Autodesk Fusion 360 part; units mm, degrees
(part 7 of 15)
  arc A95 (-74.6061, -67.9864) -> (-74.325, -69.279) centre (-2.0032, -52.8695) ccw
  spline S95 degree 5 poles (-74.325, -69.279) (-74.3068, -69.2823) (-74.2706, -69.289) (-74.2162, -69.2989) (-74.1437, -69.3119) (-74.053, -69.3279) (-73.9624, -69.3436) (-73.8718, -69.359) (-73.7813, -69.3741) (-73.6907, -69.3889) (-73.6002, -69.4033) (-73.5096, -69.4175) (-73.4191, -69.4313) (-73.3287, -69.4448) (-73.2382, -69.458) (-73.1478, -69.4709) (-73.0573, -69.4835) (-72.9669, -69.4957) (-72.8766, -69.5076) (-72.7862, -69.5192) (-72.6959, -69.5304) (-72.6056, -69.5413) (-72.5153, -69.5519) (-72.4251, -69.5621) (-72.3349, -69.572) (-72.2447, -69.5815) (-72.1546, -69.5907) (-72.0644, -69.5996) (-71.9744, -69.6081) (-71.8843, -69.6162) (-71.7943, -69.6239) (-71.7043, -69.6313) (-71.6144, -69.6384) (-71.5245, -69.645) (-71.4347, -69.6513) (-71.3449, -69.6572) (-71.2551, -69.6627) (-71.1654, -69.6678) (-71.0757, -69.6725) (-70.9861, -69.6768) (-70.8965, -69.6808) (-70.807, -69.6843) (-70.7248, -69.6871) (-70.6606, -69.689) (-70.6143, -69.6903) (-70.5859, -69.691) (-70.5753, -69.6913) knots -1 -1 -1 -1 -1 -1 -0.985714 -0.971429 -0.957143 -0.942857 -0.928571 -0.914286 -0.9 -0.885714 -0.871429 -0.857143 -0.842857 -0.828571 -0.814286 -0.8 -0.785714 -0.771429 -0.757143 -0.742857 -0.728571 -0.714286 -0.7 -0.685714 -0.671429 -0.657143 -0.642857 -0.628571 -0.614286 -0.6 -0.585714 -0.571429 -0.557143 -0.542857 -0.528571 -0.514286 -0.5 -0.485714 -0.471429 -0.457143 -0.442857 -0.428571 -0.414286 -0.405839 -0.405839 -0.405839 -0.405839 -0.405839 -0.405839
  arc A96 (-70.5753, -69.6913) -> (-70.2493, -70.9684) centre (-2.0032, -52.8695) ccw
  spline S96 degree 5 poles (-70.2493, -70.9684) (-70.2585, -70.9737) (-70.2831, -70.988) (-70.3231, -71.0113) (-70.3786, -71.0438) (-70.4493, -71.0856) (-70.5262, -71.1316) (-70.6029, -71.178) (-70.6795, -71.2247) (-70.756, -71.2718) (-70.8323, -71.3193) (-70.9084, -71.3672) (-70.9844, -71.4154) (-71.0603, -71.464) (-71.136, -71.5129) (-71.2115, -71.5621) (-71.287, -71.6118) (-71.3622, -71.6617) (-71.4374, -71.712) (-71.5124, -71.7626) (-71.5872, -71.8135) (-71.6619, -71.8648) (-71.7365, -71.9164) (-71.8109, -71.9683) (-71.8852, -72.0205) (-71.9594, -72.0731) (-72.0334, -72.1259) (-72.1073, -72.1791) (-72.1811, -72.2325) (-72.2547, -72.2863) (-72.3282, -72.3404) (-72.4015, -72.3947) (-72.4747, -72.4494) (-72.5478, -72.5043) (-72.6207, -72.5595) (-72.6935, -72.615) (-72.7662, -72.6709) (-72.8387, -72.7269) (-72.9111, -72.7833) (-72.9834, -72.8399) (-73.0555, -72.8969) (-73.1275, -72.9541) (-73.1994, -73.0115) (-73.2568, -73.0577) (-73.2998, -73.0925) (-73.3284, -73.1157) (-73.3427, -73.1273) knots 0.405839 0.405839 0.405839 0.405839 0.405839 0.405839 0.414286 0.428571 0.442857 0.457143 0.471429 0.485714 0.5 0.514286 0.528571 0.542857 0.557143 0.571429 0.585714 0.6 0.614286 0.628571 0.642857 0.657143 0.671429 0.685714 0.7 0.714286 0.728571 0.742857 0.757143 0.771429 0.785714 0.8 0.814286 0.828571 0.842857 0.857143 0.871429 0.885714 0.9 0.914286 0.928571 0.942857 0.957143 0.971429 0.985714 1 1 1 1 1 1
  arc A97 (-73.3427, -73.1273) -> (-72.97, -74.3965) centre (-2.0032, -52.8695) ccw
  spline S97 degree 5 poles (-72.97, -74.3965) (-72.9517, -74.3986) (-72.9151, -74.4026) (-72.8601, -74.4087) (-72.7869, -74.4165) (-72.6953, -74.426) (-72.6038, -74.4352) (-72.5124, -74.444) (-72.421, -74.4526) (-72.3296, -74.4609) (-72.2382, -74.4689) (-72.1469, -74.4765) (-72.0557, -74.4839) (-71.9645, -74.4909) (-71.8733, -74.4976) (-71.7822, -74.504) (-71.6911, -74.5101) (-71.6, -74.5158) (-71.509, -74.5213) (-71.4181, -74.5264) (-71.3272, -74.5311) (-71.2364, -74.5356) (-71.1456, -74.5397) (-71.0548, -74.5434) (-70.9641, -74.5469) (-70.8735, -74.5499) (-70.7829, -74.5527) (-70.6924, -74.5551) (-70.602, -74.5571) (-70.5116, -74.5588) (-70.4212, -74.5601) (-70.331, -74.5611) (-70.2408, -74.5616) (-70.1506, -74.5619) (-70.0606, -74.5617) (-69.9706, -74.5612) (-69.8806, -74.5603) (-69.7908, -74.559) (-69.701, -74.5573) (-69.6113, -74.5552) (-69.5217, -74.5527) (-69.4321, -74.5498) (-69.35, -74.5468) (-69.2858, -74.5441) (-69.2395, -74.5421) (-69.2111, -74.5408) (-69.2005, -74.5403) knots -1 -1 -1 -1 -1 -1 -0.985714 -0.971429 -0.957143 -0.942857 -0.928571 -0.914286 -0.9 -0.885714 -0.871429 -0.857143 -0.842857 -0.828571 -0.814286 -0.8 -0.785714 -0.771429 -0.757143 -0.742857 -0.728571 -0.714286 -0.7 -0.685714 -0.671429 -0.657143 -0.642857 -0.628571 -0.614286 -0.6 -0.585714 -0.571429 -0.557143 -0.542857 -0.528571 -0.514286 -0.5 -0.485714 -0.471429 -0.457143 -0.442857 -0.428571 -0.414286 -0.405839 -0.405839 -0.405839 -0.405839 -0.405839 -0.405839
  arc A98 (-69.2005, -74.5403) -> (-68.7843, -75.791) centre (-2.0032, -52.8695) ccw
  spline S98 degree 5 poles (-68.7843, -75.791) (-68.793, -75.7969) (-68.8166, -75.8129) (-68.8548, -75.839) (-68.9078, -75.8753) (-68.9754, -75.9221) (-69.0488, -75.9735) (-69.1221, -76.0252) (-69.1951, -76.0773) (-69.268, -76.1297) (-69.3407, -76.1825) (-69.4132, -76.2357) (-69.4856, -76.2892) (-69.5578, -76.3431) (-69.6298, -76.3973) (-69.7017, -76.4518) (-69.7734, -76.5066) (-69.8449, -76.5618) (-69.9163, -76.6174) (-69.9874, -76.6732) (-70.0585, -76.7293) (-70.1293, -76.7858) (-70.2, -76.8426) (-70.2706, -76.8997) (-70.341, -76.9571) (-70.4112, -77.0148) (-70.4813, -77.0728) (-70.5512, -77.131) (-70.6209, -77.1896) (-70.6905, -77.2485) (-70.7599, -77.3077) (-70.8292, -77.3671) (-70.8983, -77.4269) (-70.9673, -77.4869) (-71.0361, -77.5472) (-71.1048, -77.6077) (-71.1733, -77.6686) (-71.2416, -77.7297) (-71.3098, -77.7911) (-71.3779, -77.8527) (-71.4458, -77.9146) (-71.5135, -77.9768) (-71.5811, -78.0393) (-71.635, -78.0894) (-71.6754, -78.1272) (-71.7023, -78.1524) (-71.7158, -78.165) knots 0.405839 0.405839 0.405839 0.405839 0.405839 0.405839 0.414286 0.428571 0.442857 0.457143 0.471429 0.485714 0.5 0.514286 0.528571 0.542857 0.557143 0.571429 0.585714 0.6 0.614286 0.628571 0.642857 0.657143 0.671429 0.685714 0.7 0.714286 0.728571 0.742857 0.757143 0.771429 0.785714 0.8 0.814286 0.828571 0.842857 0.857143 0.871429 0.885714 0.9 0.914286 0.928571 0.942857 0.957143 0.971429 0.985714 1 1 1 1 1 1
  arc A99 (-71.7158, -78.165) -> (-71.2535, -79.4044) centre (-2.0032, -52.8695) ccw
  spline S99 degree 5 poles (-71.2535, -79.4044) (-71.2351, -79.4051) (-71.1982, -79.4066) (-71.143, -79.4086) (-71.0694, -79.4112) (-70.9774, -79.4142) (-70.8855, -79.4168) (-70.7936, -79.4191) (-70.7018, -79.4212) (-70.6101, -79.4229) (-70.5184, -79.4243) (-70.4268, -79.4255) (-70.3352, -79.4263) (-70.2438, -79.4268) (-70.1523, -79.427) (-70.061, -79.4268) (-69.9697, -79.4264) (-69.8785, -79.4257) (-69.7873, -79.4246) (-69.6962, -79.4232) (-69.6052, -79.4214) (-69.5143, -79.4194) (-69.4235, -79.417) (-69.3327, -79.4143) (-69.242, -79.4112) (-69.1514, -79.4079) (-69.0608, -79.4041) (-68.9704, -79.4) (-68.88, -79.3956) (-68.7897, -79.3908) (-68.6995, -79.3857) (-68.6094, -79.3802) (-68.5194, -79.3744) (-68.4295, -79.3682) (-68.3397, -79.3616) (-68.2499, -79.3547) (-68.1603, -79.3473) (-68.0708, -79.3396) (-67.9813, -79.3315) (-67.892, -79.3231) (-67.8028, -79.3142) (-67.7137, -79.3049) (-67.632, -79.296) (-67.5681, -79.2888) (-67.5221, -79.2835) (-67.4938, -79.2801) (-67.4833, -79.2789) knots -1 -1 -1 -1 -1 -1 -0.985714 -0.971429 -0.957143 -0.942857 -0.928571 -0.914286 -0.9 -0.885714 -0.871429 -0.857143 -0.842857 -0.828571 -0.814286 -0.8 -0.785714 -0.771429 -0.757143 -0.742857 -0.728571 -0.714286 -0.7 -0.685714 -0.671429 -0.657143 -0.642857 -0.628571 -0.614286 -0.6 -0.585714 -0.571429 -0.557143 -0.542857 -0.528571 -0.514286 -0.5 -0.485714 -0.471429 -0.457143 -0.442857 -0.428571 -0.414286 -0.405839 -0.405839 -0.405839 -0.405839 -0.405839 -0.405839
  arc A100 (-67.4833, -79.2789) -> (-66.9789, -80.4967) centre (-2.0032, -52.8695) ccw
  spline S100 degree 5 poles (-66.9789, -80.4967) (-66.9872, -80.5032) (-67.0096, -80.5208) (-67.0459, -80.5496) (-67.0961, -80.5896) (-67.1602, -80.6411) (-67.2298, -80.6976) (-67.2991, -80.7544) (-67.3683, -80.8116) (-67.4372, -80.8691) (-67.506, -80.9269) (-67.5746, -80.9851) (-67.6429, -81.0437) (-67.7111, -81.1025) (-67.7791, -81.1617) (-67.8469, -81.2213) (-67.9144, -81.2811) (-67.9818, -81.3412) (-68.0491, -81.4017) (-68.1161, -81.4625) (-68.1829, -81.5236) (-68.2496, -81.5849) (-68.3161, -81.6466) (-68.3824, -81.7086) (-68.4485, -81.7709) (-68.5144, -81.8334) (-68.5801, -81.8963) (-68.6457, -81.9594) (-68.7111, -82.0228) (-68.7763, -82.0865) (-68.8414, -82.1505) (-68.9062, -82.2147) (-68.9709, -82.2792) (-69.0354, -82.344) (-69.0997, -82.409) (-69.1639, -82.4743) (-69.2279, -82.5399) (-69.2917, -82.6058) (-69.3553, -82.6719) (-69.4188, -82.7382) (-69.4821, -82.8048) (-69.5453, -82.8717) (-69.6082, -82.9388) (-69.6585, -82.9927) (-69.6961, -83.0332) (-69.7211, -83.0603) (-69.7336, -83.0738) knots 0.405839 0.405839 0.405839 0.405839 0.405839 0.405839 0.414286 0.428571 0.442857 0.457143 0.471429 0.485714 0.5 0.514286 0.528571 0.542857 0.557143 0.571429 0.585714 0.6 0.614286 0.628571 0.642857 0.657143 0.671429 0.685714 0.7 0.714286 0.728571 0.742857 0.757143 0.771429 0.785714 0.8 0.814286 0.828571 0.842857 0.857143 0.871429 0.885714 0.9 0.914286 0.928571 0.942857 0.957143 0.971429 0.985714 1 1 1 1 1 1
  arc A101 (-69.7336, -83.0738) -> (-69.1841, -84.2771) centre (-2.0032, -52.8695) ccw
  spline S101 degree 5 poles (-69.1841, -84.2771) (-69.1657, -84.2765) (-69.1288, -84.2753) (-69.0736, -84.2734) (-68.9999, -84.2707) (-68.908, -84.2671) (-68.8161, -84.2632) (-68.7243, -84.2589) (-68.6326, -84.2544) (-68.541, -84.2496) (-68.4494, -84.2445) (-68.358, -84.2391) (-68.2666, -84.2334) (-68.1753, -84.2273) (-68.0841, -84.221) (-67.993, -84.2144) (-67.902, -84.2074) (-67.811, -84.2002) (-67.7202, -84.1926) (-67.6295, -84.1847) (-67.5388, -84.1765) (-67.4483, -84.1679) (-67.3578, -84.1591) (-67.2675, -84.1499) (-67.1772, -84.1404) (-67.0871, -84.1305) (-66.997, -84.1203) (-66.9071, -84.1098) (-66.8173, -84.099) (-66.7276, -84.0878) (-66.638, -84.0762) (-66.5485, -84.0643) (-66.4591, -84.0521) (-66.3698, -84.0395) (-66.2807, -84.0265) (-66.1917, -84.0132) (-66.1028, -83.9995) (-66.0141, -83.9854) (-65.9254, -83.9709) (-65.837, -83.9561) (-65.7486, -83.9409) (-65.6604, -83.9253) (-65.5795, -83.9106) (-65.5163, -83.8988) (-65.4708, -83.8902) (-65.4429, -83.8849) (-65.4325, -83.8829) knots -1 -1 -1 -1 -1 -1 -0.985714 -0.971429 -0.957143 -0.942857 -0.928571 -0.914286 -0.9 -0.885714 -0.871429 -0.857143 -0.842857 -0.828571 -0.814286 -0.8 -0.785714 -0.771429 -0.757143 -0.742857 -0.728571 -0.714286 -0.7 -0.685714 -0.671429 -0.657143 -0.642857 -0.628571 -0.614286 -0.6 -0.585714 -0.571429 -0.557143 -0.542857 -0.528571 -0.514286 -0.5 -0.485714 -0.471429 -0.457143 -0.442857 -0.428571 -0.414286 -0.405839 -0.405839 -0.405839 -0.405839 -0.405839 -0.405839
  arc A102 (-65.4325, -83.8829) -> (-64.8425, -85.0616) centre (-2.0032, -52.8695) ccw
  spline S102 degree 5 poles (-64.8425, -85.0616) (-64.8503, -85.0687) (-64.8713, -85.0879) (-64.9055, -85.1191) (-64.9528, -85.1627) (-65.013, -85.2186) (-65.0783, -85.2799) (-65.1435, -85.3415) (-65.2084, -85.4035) (-65.2731, -85.4657) (-65.3375, -85.5284) (-65.4017, -85.5913) (-65.4658, -85.6546) (-65.5296, -85.7181) (-65.5931, -85.782) (-65.6565, -85.8462) (-65.7197, -85.9108) (-65.7826, -85.9756) (-65.8453, -86.0407) (-65.9078, -86.1061) (-65.9702, -86.1718) (-66.0323, -86.2377) (-66.0942, -86.304) (-66.1559, -86.3705) (-66.2174, -86.4374) (-66.2787, -86.5045) (-66.3398, -86.5718) (-66.4007, -86.6395) (-66.4614, -86.7074) (-66.5219, -86.7756) (-66.5822, -86.844) (-66.6423, -86.9127) (-66.7022, -86.9817) (-66.7619, -87.0509) (-66.8215, -87.1204) (-66.8808, -87.1901) (-66.9399, -87.2601) (-66.9989, -87.3303) (-67.0577, -87.4008) (-67.1162, -87.4715) (-67.1746, -87.5424) (-67.2328, -87.6136) (-67.2908, -87.6851) (-67.3371, -87.7424) (-67.3717, -87.7855) (-67.3948, -87.8143) (-67.4063, -87.8287) knots 0.405839 0.405839 0.405839 0.405839 0.405839 0.405839 0.414286 0.428571 0.442857 0.457143 0.471429 0.485714 0.5 0.514286 0.528571 0.542857 0.557143 0.571429 0.585714 0.6 0.614286 0.628571 0.642857 0.657143 0.671429 0.685714 0.7 0.714286 0.728571 0.742857 0.757143 0.771429 0.785714 0.8 0.814286 0.828571 0.842857 0.857143 0.871429 0.885714 0.9 0.914286 0.928571 0.942857 0.957143 0.971429 0.985714 1 1 1 1 1 1
  arc A103 (-67.4063, -87.8287) -> (-66.7723, -88.9897) centre (-2.0032, -52.8695) ccw
  spline S103 degree 5 poles (-66.7723, -88.9897) (-66.754, -88.9878) (-66.7173, -88.9839) (-66.6623, -88.9781) (-66.5891, -88.9702) (-66.4976, -88.96) (-66.4063, -88.9496) (-66.315, -88.9388) (-66.2239, -88.9277) (-66.1328, -88.9164) (-66.0419, -88.9048) (-65.951, -88.8928) (-65.8603, -88.8806) (-65.7697, -88.8681) (-65.6791, -88.8553) (-65.5887, -88.8422) (-65.4984, -88.8287) (-65.4083, -88.815) (-65.3182, -88.801) (-65.2282, -88.7866) (-65.1384, -88.772) (-65.0487, -88.757) (-64.9591, -88.7417) (-64.8697, -88.7261) (-64.7803, -88.7102) (-64.6911, -88.6939) (-64.602, -88.6773) (-64.5131, -88.6604) (-64.4242, -88.6432) (-64.3356, -88.6256) (-64.247, -88.6077) (-64.1586, -88.5894) (-64.0703, -88.5709) (-63.9822, -88.5519) (-63.8942, -88.5326) (-63.8064, -88.513) (-63.7187, -88.493) (-63.6312, -88.4726) (-63.5438, -88.4519) (-63.4566, -88.4307) (-63.3696, -88.4093) (-63.2827, -88.3874) (-63.2031, -88.367) (-63.1409, -88.3508) (-63.0961, -88.3389) (-63.0686, -88.3316) (-63.0584, -88.3289) knots -1 -1 -1 -1 -1 -1 -0.985714 -0.971429 -0.957143 -0.942857 -0.928571 -0.914286 -0.9 -0.885714 -0.871429 -0.857143 -0.842857 -0.828571 -0.814286 -0.8 -0.785714 -0.771429 -0.757143 -0.742857 -0.728571 -0.714286 -0.7 -0.685714 -0.671429 -0.657143 -0.642857 -0.628571 -0.614286 -0.6 -0.585714 -0.571429 -0.557143 -0.542857 -0.528571 -0.514286 -0.5 -0.485714 -0.471429 -0.457143 -0.442857 -0.428571 -0.414286 -0.405839 -0.405839 -0.405839 -0.405839 -0.405839 -0.405839
  arc A104 (-63.0584, -88.3289) -> (-62.3858, -89.4625) centre (-2.0032, -52.8695) ccw
  spline S104 degree 5 poles (-62.3858, -89.4625) (-62.3931, -89.4701) (-62.4127, -89.4907) (-62.4446, -89.5244) (-62.4886, -89.5712) (-62.5447, -89.6313) (-62.6055, -89.697) (-62.6661, -89.7631) (-62.7264, -89.8296) (-62.7865, -89.8963) (-62.8463, -89.9634) (-62.9059, -90.0307) (-62.9652, -90.0984) (-63.0243, -90.1664) (-63.0832, -90.2346) (-63.1418, -90.3032) (-63.2002, -90.372) (-63.2583, -90.4412) (-63.3163, -90.5106) (-63.374, -90.5803) (-63.4314, -90.6503) (-63.4887, -90.7205) (-63.5457, -90.791) (-63.6025, -90.8618) (-63.6591, -90.9328) (-63.7154, -91.0041) (-63.7715, -91.0757) (-63.8275, -91.1475) (-63.8832, -91.2196) (-63.9386, -91.2919) (-63.9939, -91.3645) (-64.049, -91.4373) (-64.1038, -91.5103) (-64.1585, -91.5837) (-64.2129, -91.6572) (-64.2671, -91.731) (-64.3211, -91.805) (-64.3749, -91.8792) (-64.4285, -91.9537) (-64.4819, -92.0284) (-64.535, -92.1034) (-64.588, -92.1785) (-64.6408, -92.2539) (-64.6828, -92.3144) (-64.7143, -92.3599) (-64.7352, -92.3902) (-64.7457, -92.4054) knots 0.405839 0.405839 0.405839 0.405839 0.405839 0.405839 0.414286 0.428571 0.442857 0.457143 0.471429 0.485714 0.5 0.514286 0.528571 0.542857 0.557143 0.571429 0.585714 0.6 0.614286 0.628571 0.642857 0.657143 0.671429 0.685714 0.7 0.714286 0.728571 0.742857 0.757143 0.771429 0.785714 0.8 0.814286 0.828571 0.842857 0.857143 0.871429 0.885714 0.9 0.914286 0.928571 0.942857 0.957143 0.971429 0.985714 1 1 1 1 1 1
  arc A105 (-64.7457, -92.4054) -> (-64.0305, -93.5182) centre (-2.0032, -52.8695) ccw
  spline S105 degree 5 poles (-64.0305, -93.5182) (-64.0124, -93.515) (-63.9761, -93.5086) (-63.9216, -93.4989) (-63.8491, -93.4857) (-63.7586, -93.4691) (-63.6683, -93.4521) (-63.578, -93.4348) (-63.4879, -93.4173) (-63.3979, -93.3995) (-63.308, -93.3814) (-63.2182, -93.363) (-63.1286, -93.3444) (-63.0391, -93.3254) (-62.9497, -93.3062) (-62.8605, -93.2866) (-62.7714, -93.2668) (-62.6824, -93.2467) (-62.5936, -93.2263) (-62.5049, -93.2055) (-62.4163, -93.1845) (-62.3279, -93.1632) (-62.2396, -93.1415) (-62.1515, -93.1196) (-62.0635, -93.0973) (-61.9757, -93.0747) (-61.888, -93.0518) (-61.8005, -93.0286) (-61.7131, -93.0051) (-61.6259, -92.9812) (-61.5389, -92.9571) (-61.452, -92.9325) (-61.3653, -92.9077) (-61.2787, -92.8825) (-61.1924, -92.857) (-61.1062, -92.8311) (-61.0201, -92.8049) (-60.9343, -92.7784) (-60.8486, -92.7515) (-60.7631, -92.7242) (-60.6778, -92.6965) (-60.5927, -92.6685) (-60.5148, -92.6425) (-60.4539, -92.6219) (-60.4101, -92.6069) (-60.3832, -92.5976) (-60.3732, -92.5941) knots -1 -1 -1 -1 -1 -1 -0.985714 -0.971429 -0.957143 -0.942857 -0.928571 -0.914286 -0.9 -0.885714 -0.871429 -0.857143 -0.842857 -0.828571 -0.814286 -0.8 -0.785714 -0.771429 -0.757143 -0.742857 -0.728571 -0.714286 -0.7 -0.685714 -0.671429 -0.657143 -0.642857 -0.628571 -0.614286 -0.6 -0.585714 -0.571429 -0.557143 -0.542857 -0.528571 -0.514286 -0.5 -0.485714 -0.471429 -0.457143 -0.442857 -0.428571 -0.414286 -0.405839 -0.405839 -0.405839 -0.405839 -0.405839 -0.405839
  arc A106 (-60.3732, -92.5941) -> (-59.6214, -93.6769) centre (-2.0032, -52.8695) ccw
  spline S106 degree 5 poles (-59.6214, -93.6769) (-59.6282, -93.685) (-59.6462, -93.707) (-59.6756, -93.7428) (-59.7162, -93.7926) (-59.7679, -93.8566) (-59.8238, -93.9265) (-59.8795, -93.9968) (-59.935, -94.0673) (-59.9901, -94.1382) (-60.045, -94.2093) (-60.0996, -94.2808) (-60.154, -94.3525) (-60.2081, -94.4245) (-60.2619, -94.4968) (-60.3155, -94.5694) (-60.3688, -94.6422) (-60.4219, -94.7153) (-60.4747, -94.7887) (-60.5273, -94.8623) (-60.5797, -94.9362) (-60.6317, -95.0104) (-60.6836, -95.0848) (-60.7352, -95.1594) (-60.7866, -95.2343) (-60.8377, -95.3095) (-60.8886, -95.3849) (-60.9392, -95.4605) (-60.9896, -95.5363) (-61.0398, -95.6124) (-61.0898, -95.6888) (-61.1395, -95.7653) (-61.189, -95.8421) (-61.2383, -95.9191) (-61.2873, -95.9964) (-61.3361, -96.0738) (-61.3847, -96.1515) (-61.4331, -96.2294) (-61.4812, -96.3075) (-61.5291, -96.3858) (-61.5768, -96.4644) (-61.6243, -96.5431) (-61.6715, -96.6221) (-61.7092, -96.6854) (-61.7373, -96.733) (-61.756, -96.7648) (-61.7653, -96.7807) knots 0.405839 0.405839 0.405839 0.405839 0.405839 0.405839 0.414286 0.428571 0.442857 0.457143 0.471429 0.485714 0.5 0.514286 0.528571 0.542857 0.557143 0.571429 0.585714 0.6 0.614286 0.628571 0.642857 0.657143 0.671429 0.685714 0.7 0.714286 0.728571 0.742857 0.757143 0.771429 0.785714 0.8 0.814286 0.828571 0.842857 0.857143 0.871429 0.885714 0.9 0.914286 0.928571 0.942857 0.957143 0.971429 0.985714 1 1 1 1 1 1
  arc A107 (-61.7653, -96.7807) -> (-60.9726, -97.8396) centre (-2.0032, -52.8695) ccw
  spline S107 degree 5 poles (-60.9726, -97.8396) (-60.9548, -97.8351) (-60.919, -97.8261) (-60.8654, -97.8126) (-60.794, -97.7943) (-60.705, -97.7712) (-60.616, -97.7478) (-60.5272, -97.7242) (-60.4386, -97.7003) (-60.3501, -97.6761) (-60.2617, -97.6516) (-60.1735, -97.6269) (-60.0854, -97.6019) (-59.9975, -97.5766) (-59.9097, -97.551) (-59.8221, -97.5252) (-59.7346, -97.499) (-59.6473, -97.4726) (-59.5602, -97.4459) (-59.4732, -97.4189) (-59.3863, -97.3916) (-59.2997, -97.364) (-59.2132, -97.3361) (-59.1268, -97.3079) (-59.0407, -97.2795) (-58.9547, -97.2507) (-58.8689, -97.2216) (-58.7832, -97.1922) (-58.6978, -97.1625) (-58.6125, -97.1325) (-58.5274, -97.1021) (-58.4425, -97.0715) (-58.3577, -97.0405) (-58.2732, -97.0092) (-58.1889, -96.9776) (-58.1047, -96.9457) (-58.0208, -96.9134) (-57.9371, -96.8808) (-57.8535, -96.8478) (-57.7702, -96.8145) (-57.6871, -96.7809) (-57.6042, -96.7469) (-57.5283, -96.7153) (-57.4691, -96.6904) (-57.4264, -96.6723) (-57.4003, -96.6611) (-57.3905, -96.657) knots -1 -1 -1 -1 -1 -1 -0.985714 -0.971429 -0.957143 -0.942857 -0.928571 -0.914286 -0.9 -0.885714 -0.871429 -0.857143 -0.842857 -0.828571 -0.814286 -0.8 -0.785714 -0.771429 -0.757143 -0.742857 -0.728571 -0.714286 -0.7 -0.685714 -0.671429 -0.657143 -0.642857 -0.628571 -0.614286 -0.6 -0.585714 -0.571429 -0.557143 -0.542857 -0.528571 -0.514286 -0.5 -0.485714 -0.471429 -0.457143 -0.442857 -0.428571 -0.414286 -0.405839 -0.405839 -0.405839 -0.405839 -0.405839 -0.405839
  arc A108 (-57.3905, -96.657) -> (-56.5635, -97.6833) centre (-2.0032, -52.8695) ccw
  spline S108 degree 5 poles (-56.5635, -97.6833) (-56.5696, -97.6919) (-56.5861, -97.7151) (-56.6128, -97.753) (-56.6497, -97.8056) (-56.6967, -97.873) (-56.7476, -97.9468) (-56.7981, -98.0208) (-56.8484, -98.0952) (-56.8983, -98.1698) (-56.948, -98.2447) (-56.9974, -98.3198) (-57.0465, -98.3953) (-57.0953, -98.4709) (-57.1438, -98.5469) (-57.1921, -98.6231) (-57.2401, -98.6996) (-57.2878, -98.7763) (-57.3353, -98.8532) (-57.3825, -98.9304) (-57.4294, -99.0078) (-57.4761, -99.0855) (-57.5225, -99.1634) (-57.5686, -99.2416) (-57.6145, -99.3199) (-57.6601, -99.3985) (-57.7055, -99.4774) (-57.7507, -99.5564) (-57.7955, -99.6357) (-57.8402, -99.7152) (-57.8845, -99.7948) (-57.9287, -99.8748) (-57.9726, -99.9549) (-58.0162, -100.0352) (-58.0596, -100.1157) (-58.1028, -100.1965) (-58.1457, -100.2774) (-58.1884, -100.3586) (-58.2308, -100.4399) (-58.273, -100.5215) (-58.315, -100.6032) (-58.3567, -100.6852) (-58.3982, -100.7673) (-58.4313, -100.8331) (-58.4559, -100.8826) (-58.4723, -100.9157) (-58.4805, -100.9322) knots 0.405839 0.405839 0.405839 0.405839 0.405839 0.405839 0.414286 0.428571 0.442857 0.457143 0.471429 0.485714 0.5 0.514286 0.528571 0.542857 0.557143 0.571429 0.585714 0.6 0.614286 0.628571 0.642857 0.657143 0.671429 0.685714 0.7 0.714286 0.728571 0.742857 0.757143 0.771429 0.785714 0.8 0.814286 0.828571 0.842857 0.857143 0.871429 0.885714 0.9 0.914286 0.928571 0.942857 0.957143 0.971429 0.985714 1 1 1 1 1 1
  arc A109 (-58.4805, -100.9322) -> (-57.6143, -101.9319) centre (-2.0032, -52.8695) ccw
  spline S109 degree 5 poles (-57.6143, -101.9319) (-57.5967, -101.9261) (-57.5617, -101.9146) (-57.5092, -101.8972) (-57.4393, -101.8739) (-57.3521, -101.8445) (-57.2651, -101.8149) (-57.1782, -101.785) (-57.0915, -101.7548) (-57.0049, -101.7243) (-56.9185, -101.6936) (-56.8323, -101.6627) (-56.7462, -101.6315) (-56.6603, -101.6) (-56.5746, -101.5682) (-56.4891, -101.5361) (-56.4037, -101.5038) (-56.3185, -101.4712) (-56.2335, -101.4384) (-56.1486, -101.4052) (-56.064, -101.3718) (-55.9795, -101.3381) (-55.8952, -101.3041) (-55.8111, -101.2699) (-55.7272, -101.2353) (-55.6435, -101.2005) (-55.5599, -101.1653) (-55.4766, -101.1299) (-55.3935, -101.0942) (-55.3106, -101.0582) (-55.2278, -101.0218) (-55.1453, -100.9852) (-55.063, -100.9483) (-54.9809, -100.911) (-54.8991, -100.8735) (-54.8174, -100.8356) (-54.736, -100.7974) (-54.6548, -100.7589) (-54.5739, -100.7201) (-54.4931, -100.6809) (-54.4126, -100.6414) (-54.3324, -100.6016) (-54.2589, -100.5647) (-54.2016, -100.5356) (-54.1604, -100.5146) (-54.1351, -100.5016) (-54.1257, -100.4967) knots -1 -1 -1 -1 -1 -1 -0.985714 -0.971429 -0.957143 -0.942857 -0.928571 -0.914286 -0.9 -0.885714 -0.871429 -0.857143 -0.842857 -0.828571 -0.814286 -0.8 -0.785714 -0.771429 -0.757143 -0.742857 -0.728571 -0.714286 -0.7 -0.685714 -0.671429 -0.657143 -0.642857 -0.628571 -0.614286 -0.6 -0.585714 -0.571429 -0.557143 -0.542857 -0.528571 -0.514286 -0.5 -0.485714 -0.471429 -0.457143 -0.442857 -0.428571 -0.414286 -0.405839 -0.405839 -0.405839 -0.405839 -0.405839 -0.405839
  arc A110 (-54.1257, -100.4967) -> (-53.2275, -101.4614) centre (-2.0032, -52.8695) ccw
  spline S110 degree 5 poles (-53.2275, -101.4614) (-53.233, -101.4705) (-53.2477, -101.4948) (-53.2717, -101.5344) (-53.3048, -101.5895) (-53.3468, -101.6602) (-53.3923, -101.7374) (-53.4374, -101.8148) (-53.4822, -101.8926) (-53.5268, -101.9705) (-53.571, -102.0488) (-53.6149, -102.1273) (-53.6585, -102.206) (-53.7018, -102.285) (-53.7448, -102.3642) (-53.7875, -102.4437) (-53.8299, -102.5233) (-53.872, -102.6033) (-53.9139, -102.6834) (-53.9554, -102.7638) (-53.9967, -102.8444) (-54.0377, -102.9252) (-54.0784, -103.0062) (-54.1189, -103.0874) (-54.1591, -103.1689) (-54.199, -103.2505) (-54.2386, -103.3324) (-54.278, -103.4144) (-54.3171, -103.4967) (-54.356, -103.5792) (-54.3945, -103.6618) (-54.4329, -103.7447) (-54.4709, -103.8277) (-54.5087, -103.911) (-54.5463, -103.9944) (-54.5836, -104.078) (-54.6206, -104.1618) (-54.6574, -104.2458) (-54.6939, -104.33) (-54.7302, -104.4143) (-54.7662, -104.4988) (-54.802, -104.5835) (-54.8376, -104.6684) (-54.8658, -104.7365) (-54.8869, -104.7876) (-54.9009, -104.8217) (-54.9078, -104.8388) knots 0.405839 0.405839 0.405839 0.405839 0.405839 0.405839 0.414286 0.428571 0.442857 0.457143 0.471429 0.485714 0.5 0.514286 0.528571 0.542857 0.557143 0.571429 0.585714 0.6 0.614286 0.628571 0.642857 0.657143 0.671429 0.685714 0.7 0.714286 0.728571 0.742857 0.757143 0.771429 0.785714 0.8 0.814286 0.828571 0.842857 0.857143 0.871429 0.885714 0.9 0.914286 0.928571 0.942857 0.957143 0.971429 0.985714 1 1 1 1 1 1
  arc A111 (-54.9078, -104.8388) -> (-53.9725, -105.7741) centre (-2.0032, -52.8695) ccw
  spline S111 degree 5 poles (-53.9725, -105.7741) (-53.9554, -105.7671) (-53.9213, -105.7531) (-53.8702, -105.7321) (-53.8022, -105.7038) (-53.7173, -105.6683) (-53.6326, -105.6325) (-53.548, -105.5965) (-53.4637, -105.5602) (-53.3795, -105.5236) (-53.2955, -105.4869) (-53.2117, -105.4498) (-53.1281, -105.4125) (-53.0447, -105.375) (-52.9615, -105.3372) (-52.8784, -105.2991) (-52.7955, -105.2608) (-52.7129, -105.2222) (-52.6304, -105.1834) (-52.5482, -105.1443) (-52.4661, -105.1049) (-52.3842, -105.0653) (-52.3026, -105.0253) (-52.2211, -104.9852) (-52.1399, -104.9447) (-52.0589, -104.904) (-51.9781, -104.863) (-51.8975, -104.8217) (-51.8171, -104.7801) (-51.737, -104.7383) (-51.6571, -104.6962) (-51.5774, -104.6537) (-51.4979, -104.611) (-51.4187, -104.568) (-51.3397, -104.5247) (-51.261, -104.4811) (-51.1825, -104.4372) (-51.1043, -104.393) (-51.0263, -104.3485) (-50.9486, -104.3037) (-50.8711, -104.2586) (-50.7939, -104.2131) (-50.7232, -104.1711) (-50.6682, -104.138) (-50.6285, -104.114) (-50.6042, -104.0992) (-50.5952, -104.0937) knots -1 -1 -1 -1 -1 -1 -0.985714 -0.971429 -0.957143 -0.942857 -0.928571 -0.914286 -0.9 -0.885714 -0.871429 -0.857143 -0.842857 -0.828571 -0.814286 -0.8 -0.785714 -0.771429 -0.757143 -0.742857 -0.728571 -0.714286 -0.7 -0.685714 -0.671429 -0.657143 -0.642857 -0.628571 -0.614286 -0.6 -0.585714 -0.571429 -0.557143 -0.542857 -0.528571 -0.514286 -0.5 -0.485714 -0.471429 -0.457143 -0.442857 -0.428571 -0.414286 -0.405839 -0.405839 -0.405839 -0.405839 -0.405839 -0.405839
  arc A112 (-50.5952, -104.0937) -> (-49.6305, -104.9919) centre (-2.0032, -52.8695) ccw
  spline S112 degree 5 poles (-49.6305, -104.9919) (-49.6353, -105.0013) (-49.6483, -105.0266) (-49.6694, -105.0679) (-49.6985, -105.1252) (-49.7353, -105.1987) (-49.7752, -105.2789) (-49.8147, -105.3594) (-49.8538, -105.4401) (-49.8927, -105.5211) (-49.9312, -105.6023) (-49.9693, -105.6837) (-50.0072, -105.7653) (-50.0448, -105.8472) (-50.082, -105.9293) (-50.1189, -106.0116) (-50.1556, -106.0941) (-50.1919, -106.1768) (-50.2279, -106.2597) (-50.2636, -106.3429) (-50.2991, -106.4262) (-50.3342, -106.5097) (-50.3691, -106.5934) (-50.4036, -106.6774) (-50.4379, -106.7615) (-50.4719, -106.8457) (-50.5056, -106.9302) (-50.539, -107.0149) (-50.5721, -107.0997) (-50.605, -107.1848) (-50.6376, -107.27) (-50.6699, -107.3553) (-50.7019, -107.4409) (-50.7337, -107.5266) (-50.7652, -107.6125) (-50.7964, -107.6986) (-50.8274, -107.7848) (-50.8581, -107.8712) (-50.8885, -107.9578) (-50.9187, -108.0445) (-50.9486, -108.1314) (-50.9783, -108.2184) (-51.0077, -108.3056) (-51.031, -108.3755) (-51.0483, -108.428) (-51.0598, -108.463) (-51.0656, -108.4805) knots 0.405839 0.405839 0.405839 0.405839 0.405839 0.405839 0.414286 0.428571 0.442857 0.457143 0.471429 0.485714 0.5 0.514286 0.528571 0.542857 0.557143 0.571429 0.585714 0.6 0.614286 0.628571 0.642857 0.657143 0.671429 0.685714 0.7 0.714286 0.728571 0.742857 0.757143 0.771429 0.785714 0.8 0.814286 0.828571 0.842857 0.857143 0.871429 0.885714 0.9 0.914286 0.928571 0.942857 0.957143 0.971429 0.985714 1 1 1 1 1 1
  arc A113 (-51.0656, -108.4805) -> (-50.0659, -109.3468) centre (-2.0032, -52.8695) ccw
  spline S113 degree 5 poles (-50.0659, -109.3468) (-50.0494, -109.3386) (-50.0164, -109.3222) (-49.9669, -109.2975) (-49.901, -109.2645) (-49.8189, -109.223) (-49.737, -109.1813) (-49.6552, -109.1393) (-49.5737, -109.0971) (-49.4923, -109.0546) (-49.4112, -109.012) (-49.3302, -108.969) (-49.2495, -108.9259) (-49.1689, -108.8825) (-49.0886, -108.8388) (-49.0085, -108.7949) (-48.9286, -108.7508) (-48.8489, -108.7064) (-48.7694, -108.6618) (-48.6901, -108.6169) (-48.6111, -108.5718) (-48.5323, -108.5264) (-48.4537, -108.4808) (-48.3753, -108.4349) (-48.2972, -108.3887) (-48.2193, -108.3423) (-48.1416, -108.2957) (-48.0641, -108.2487) (-47.987, -108.2016) (-47.91, -108.1541) (-47.8333, -108.1064) (-47.7568, -108.0584) (-47.6806, -108.0101) (-47.6047, -107.9616) (-47.529, -107.9127) (-47.4536, -107.8636) (-47.3784, -107.8142) (-47.3035, -107.7646) (-47.2289, -107.7146) (-47.1546, -107.6644) (-47.0805, -107.6138) (-47.0068, -107.563) (-46.9393, -107.516) (-46.8867, -107.4791) (-46.8489, -107.4523) (-46.8257, -107.4359) (-46.8171, -107.4297) knots -1 -1 -1 -1 -1 -1 -0.985714 -0.971429 -0.957143 -0.942857 -0.928571 -0.914286 -0.9 -0.885714 -0.871429 -0.857143 -0.842857 -0.828571 -0.814286 -0.8 -0.785714 -0.771429 -0.757143 -0.742857 -0.728571 -0.714286 -0.7 -0.685714 -0.671429 -0.657143 -0.642857 -0.628571 -0.614286 -0.6 -0.585714 -0.571429 -0.557143 -0.542857 -0.528571 -0.514286 -0.5 -0.485714 -0.471429 -0.457143 -0.442857 -0.428571 -0.414286 -0.405839 -0.405839 -0.405839 -0.405839 -0.405839 -0.405839
  arc A114 (-46.8171, -107.4297) -> (-45.7907, -108.2568) centre (-2.0032, -52.8695) ccw
  spline S114 degree 5 poles (-45.7907, -108.2568) (-45.7949, -108.2665) (-45.806, -108.2927) (-45.8241, -108.3354) (-45.849, -108.3946) (-45.8806, -108.4705) (-45.9146, -108.5534) (-45.9483, -108.6365) (-45.9816, -108.7198) (-46.0145, -108.8033) (-46.0471, -108.8871) (-46.0794, -108.971) (-46.1114, -109.0551) (-46.143, -109.1395) (-46.1743, -109.224) (-46.2052, -109.3087) (-46.2359, -109.3936) (-46.2662, -109.4787) (-46.2962, -109.564) (-46.3259, -109.6495) (-46.3553, -109.7351) (-46.3844, -109.8209) (-46.4132, -109.9069) (-46.4417, -109.9931) (-46.4699, -110.0794) (-46.4977, -110.1659) (-46.5253, -110.2526) (-46.5526, -110.3394) (-46.5796, -110.4264) (-46.6063, -110.5136) (-46.6328, -110.6009) (-46.6589, -110.6884) (-46.6848, -110.776) (-46.7103, -110.8637) (-46.7356, -110.9517) (-46.7606, -111.0397) (-46.7854, -111.128) (-46.8098, -111.2163) (-46.834, -111.3048) (-46.8579, -111.3935) (-46.8816, -111.4823) (-46.9049, -111.5712) (-46.928, -111.6603) (-46.9463, -111.7317) (-46.9599, -111.7853) (-46.9689, -111.821) (-46.9733, -111.8389) knots 0.405839 0.405839 0.405839 0.405839 0.405839 0.405839 0.414286 0.428571 0.442857 0.457143 0.471429 0.485714 0.5 0.514286 0.528571 0.542857 0.557143 0.571429 0.585714 0.6 0.614286 0.628571 0.642857 0.657143 0.671429 0.685714 0.7 0.714286 0.728571 0.742857 0.757143 0.771429 0.785714 0.8 0.814286 0.828571 0.842857 0.857143 0.871429 0.885714 0.9 0.914286 0.928571 0.942857 0.957143 0.971429 0.985714 1 1 1 1 1 1
  arc A115 (-46.9733, -111.8389) -> (-45.9144, -112.6316) centre (-2.0032, -52.8695) ccw
  spline S115 degree 5 poles (-45.9144, -112.6316) (-45.8985, -112.6223) (-45.8667, -112.6036) (-45.8191, -112.5754) (-45.7558, -112.5378) (-45.6769, -112.4906) (-45.5981, -112.4431) (-45.5196, -112.3954) (-45.4412, -112.3475) (-45.3631, -112.2993) (-45.2852, -112.251) (-45.2075, -112.2024) (-45.1301, -112.1536) (-45.0529, -112.1045) (-44.9758, -112.0553) (-44.8991, -112.0058) (-44.8225, -111.956) (-44.7462, -111.9061) (-44.6701, -111.8559) (-44.5942, -111.8055) (-44.5186, -111.7548) (-44.4432, -111.7039) (-44.3681, -111.6528) (-44.2932, -111.6015) (-44.2185, -111.5499) (-44.1441, -111.498) (-44.07, -111.4459) (-43.9961, -111.3936) (-43.9224, -111.341) (-43.8491, -111.2882) (-43.776, -111.2351) (-43.7031, -111.1818) (-43.6306, -111.1282) (-43.5583, -111.0744) (-43.4863, -111.0203) (-43.4145, -110.9659) (-43.3431, -110.9113) (-43.2719, -110.8564) (-43.2011, -110.8012) (-43.1305, -110.7458) (-43.0603, -110.6901) (-42.9903, -110.6341) (-42.9264, -110.5825) (-42.8766, -110.5419) (-42.8407, -110.5125) (-42.8188, -110.4944) (-42.8106, -110.4877) knots -1 -1 -1 -1 -1 -1 -0.985714 -0.971429 -0.957143 -0.942857 -0.928571 -0.914286 -0.9 -0.885714 -0.871429 -0.857143 -0.842857 -0.828571 -0.814286 -0.8 -0.785714 -0.771429 -0.757143 -0.742857 -0.728571 -0.714286 -0.7 -0.685714 -0.671429 -0.657143 -0.642857 -0.628571 -0.614286 -0.6 -0.585714 -0.571429 -0.557143 -0.542857 -0.528571 -0.514286 -0.5 -0.485714 -0.471429 -0.457143 -0.442857 -0.428571 -0.414286 -0.405839 -0.405839 -0.405839 -0.405839 -0.405839 -0.405839
  arc A116 (-42.8106, -110.4877) -> (-41.7279, -111.2395) centre (-2.0032, -52.8695) ccw
  spline S116 degree 5 poles (-41.7279, -111.2395) (-41.7313, -111.2494) (-41.7406, -111.2763) (-41.7556, -111.3202) (-41.7762, -111.381) (-41.8023, -111.459) (-41.8303, -111.5441) (-41.8579, -111.6294) (-41.8852, -111.7149) (-41.9121, -111.8005) (-41.9387, -111.8864) (-41.9649, -111.9724) (-41.9907, -112.0586) (-42.0163, -112.145) (-42.0414, -112.2316) (-42.0663, -112.3183) (-42.0908, -112.4051) (-42.115, -112.4922) (-42.1388, -112.5794) (-42.1624, -112.6668) (-42.1856, -112.7543) (-42.2085, -112.842) (-42.231, -112.9298) (-42.2533, -113.0178) (-42.2753, -113.1059) (-42.2969, -113.1942) (-42.3182, -113.2826) (-42.3393, -113.3711) (-42.36, -113.4598) (-42.3804, -113.5487) (-42.4005, -113.6376) (-42.4204, -113.7267) (-42.4399, -113.816) (-42.4592, -113.9054) (-42.4781, -113.9949) (-42.4968, -114.0845) (-42.5152, -114.1742) (-42.5332, -114.2641) (-42.5511, -114.3541) (-42.5686, -114.4443) (-42.5858, -114.5345) (-42.6028, -114.6249) (-42.6195, -114.7154) (-42.6326, -114.7879) (-42.6423, -114.8423) (-42.6487, -114.8786) (-42.6519, -114.8968) knots 0.405839 0.405839 0.405839 0.405839 0.405839 0.405839 0.414286 0.428571 0.442857 0.457143 0.471429 0.485714 0.5 0.514286 0.528571 0.542857 0.557143 0.571429 0.585714 0.6 0.614286 0.628571 0.642857 0.657143 0.671429 0.685714 0.7 0.714286 0.728571 0.742857 0.757143 0.771429 0.785714 0.8 0.814286 0.828571 0.842857 0.857143 0.871429 0.885714 0.9 0.914286 0.928571 0.942857 0.957143 0.971429 0.985714 1 1 1 1 1 1
  arc A117 (-42.6519, -114.8968) -> (-41.5391, -115.6119) centre (-2.0032, -52.8695) ccw
  spline S117 degree 5 poles (-41.5391, -115.6119) (-41.524, -115.6015) (-41.4936, -115.5806) (-41.4481, -115.5491) (-41.3876, -115.5071) (-41.3123, -115.4543) (-41.2371, -115.4013) (-41.1622, -115.3481) (-41.0875, -115.2947) (-41.013, -115.2412) (-40.9387, -115.1874) (-40.8647, -115.1334) (-40.7909, -115.0791) (-40.7174, -115.0247) (-40.6441, -114.9701) (-40.571, -114.9152) (-40.4982, -114.8602) (-40.4256, -114.8049) (-40.3533, -114.7494) (-40.2812, -114.6937) (-40.2094, -114.6378) (-40.1379, -114.5817) (-40.0666, -114.5253) (-39.9955, -114.4687) (-39.9247, -114.412) (-39.8542, -114.3549) (-39.784, -114.2977) (-39.714, -114.2402) (-39.6443, -114.1825) (-39.5749, -114.1246) (-39.5058, -114.0664) (-39.4369, -114.008) (-39.3684, -113.9494) (-39.3001, -113.8906) (-39.2321, -113.8315) (-39.1645, -113.7721) (-39.0971, -113.7126) (-39.03, -113.6527) (-38.9633, -113.5927) (-38.8969, -113.5323) (-38.8308, -113.4718) (-38.765, -113.4109) (-38.7049, -113.3549) (-38.6581, -113.3108) (-38.6245, -113.279) (-38.6038, -113.2594) (-38.5962, -113.2521) knots -1 -1 -1 -1 -1 -1 -0.985714 -0.971429 -0.957143 -0.942857 -0.928571 -0.914286 -0.9 -0.885714 -0.871429 -0.857143 -0.842857 -0.828571 -0.814286 -0.8 -0.785714 -0.771429 -0.757143 -0.742857 -0.728571 -0.714286 -0.7 -0.685714 -0.671429 -0.657143 -0.642857 -0.628571 -0.614286 -0.6 -0.585714 -0.571429 -0.557143 -0.542857 -0.528571 -0.514286 -0.5 -0.485714 -0.471429 -0.457143 -0.442857 -0.428571 -0.414286 -0.405839 -0.405839 -0.405839 -0.405839 -0.405839 -0.405839
  arc A118 (-38.5962, -113.2521) -> (-37.4626, -113.9247) centre (-2.0032, -52.8695) ccw
  spline S118 degree 5 poles (-37.4626, -113.9247) (-37.4653, -113.9349) (-37.4726, -113.9624) (-37.4845, -114.0072) (-37.5007, -114.0693) (-37.5211, -114.149) (-37.543, -114.2358) (-37.5645, -114.3229) (-37.5856, -114.4101) (-37.6063, -114.4975) (-37.6267, -114.585) (-37.6467, -114.6727) (-37.6663, -114.7605) (-37.6856, -114.8485) (-37.7046, -114.9366) (-37.7232, -115.0249) (-37.7414, -115.1133) (-37.7593, -115.2018) (-37.7769, -115.2905) (-37.7942, -115.3793) (-37.8111, -115.4683) (-37.8276, -115.5574) (-37.8439, -115.6466) (-37.8598, -115.7359) (-37.8754, -115.8254) (-37.8907, -115.915) (-37.9057, -116.0047) (-37.9204, -116.0945) (-37.9347, -116.1845) (-37.9487, -116.2745) (-37.9625, -116.3647) (-37.9759, -116.455) (-37.989, -116.5454) (-38.0018, -116.6359) (-38.0144, -116.7266) (-38.0266, -116.8173) (-38.0385, -116.9081) (-38.0501, -116.9991) (-38.0615, -117.0901) (-38.0725, -117.1813) (-38.0833, -117.2726) (-38.0938, -117.3639) (-38.1039, -117.4554) (-38.1119, -117.5286) (-38.1177, -117.5836) (-38.1215, -117.6203) (-38.1234, -117.6386) knots 0.405839 0.405839 0.405839 0.405839 0.405839 0.405839 0.414286 0.428571 0.442857 0.457143 0.471429 0.485714 0.5 0.514286 0.528571 0.542857 0.557143 0.571429 0.585714 0.6 0.614286 0.628571 0.642857 0.657143 0.671429 0.685714 0.7 0.714286 0.728571 0.742857 0.757143 0.771429 0.785714 0.8 0.814286 0.828571 0.842857 0.857143 0.871429 0.885714 0.9 0.914286 0.928571 0.942857 0.957143 0.971429 0.985714 1 1 1 1 1 1
  arc A119 (-38.1234, -117.6386) -> (-36.9624, -118.2725) centre (-2.0032, -52.8695) ccw
  spline S119 degree 5 poles (-36.9624, -118.2725) (-36.948, -118.261) (-36.9192, -118.238) (-36.8761, -118.2034) (-36.8188, -118.1571) (-36.7474, -118.0991) (-36.6762, -118.0409) (-36.6052, -117.9825) (-36.5345, -117.9239) (-36.464, -117.8652) (-36.3938, -117.8062) (-36.3238, -117.7471) (-36.2541, -117.6877) (-36.1846, -117.6282) (-36.1154, -117.5685) (-36.0465, -117.5086) (-35.9778, -117.4484) (-35.9093, -117.3881) (-35.8411, -117.3276) (-35.7732, -117.2669) (-35.7056, -117.206) (-35.6382, -117.1449) (-35.5711, -117.0836) (-35.5043, -117.0221) (-35.4377, -116.9604) (-35.3715, -116.8985) (-35.3055, -116.8364) (-35.2398, -116.7741) (-35.1744, -116.7116) (-35.1093, -116.6489) (-35.0445, -116.5859) (-34.98, -116.5228) (-34.9158, -116.4594) (-34.8519, -116.3958) (-34.7883, -116.332) (-34.725, -116.268) (-34.6621, -116.2038) (-34.5995, -116.1393) (-34.5372, -116.0746) (-34.4752, -116.0097) (-34.4136, -115.9446) (-34.3524, -115.8792) (-34.2964, -115.819) (-34.2529, -115.7718) (-34.2216, -115.7376) (-34.2024, -115.7166) (-34.1953, -115.7087) knots -1 -1 -1 -1 -1 -1 -0.985714 -0.971429 -0.957143 -0.942857 -0.928571 -0.914286 -0.9 -0.885714 -0.871429 -0.857143 -0.842857 -0.828571 -0.814286 -0.8 -0.785714 -0.771429 -0.757143 -0.742857 -0.728571 -0.714286 -0.7 -0.685714 -0.671429 -0.657143 -0.642857 -0.628571 -0.614286 -0.6 -0.585714 -0.571429 -0.557143 -0.542857 -0.528571 -0.514286 -0.5 -0.485714 -0.471429 -0.457143 -0.442857 -0.428571 -0.414286 -0.405839 -0.405839 -0.405839 -0.405839 -0.405839 -0.405839
  arc A120 (-34.1953, -115.7087) -> (-33.0166, -116.2987) centre (-2.0032, -52.8695) ccw
  spline S120 degree 5 poles (-33.0166, -116.2987) (-33.0186, -116.3091) (-33.024, -116.3371) (-33.0326, -116.3826) (-33.0443, -116.4458) (-33.059, -116.5266) (-33.0746, -116.6149) (-33.0898, -116.7032) (-33.1047, -116.7917) (-33.1191, -116.8803) (-33.1332, -116.9691) (-33.1469, -117.058) (-33.1602, -117.147) (-33.1732, -117.2361) (-33.1858, -117.3254) (-33.1981, -117.4147) (-33.21, -117.5042) (-33.2215, -117.5938) (-33.2327, -117.6835) (-33.2436, -117.7734) (-33.2541, -117.8633) (-33.2643, -117.9533) (-33.2741, -118.0435) (-33.2836, -118.1337) (-33.2928, -118.2241) (-33.3017, -118.3145) (-33.3102, -118.4051) (-33.3184, -118.4957) (-33.3263, -118.5865) (-33.3339, -118.6773) (-33.3412, -118.7682) (-33.3481, -118.8593) (-33.3547, -118.9504) (-33.3611, -119.0416) (-33.3671, -119.1329) (-33.3728, -119.2242) (-33.3782, -119.3157) (-33.3833, -119.4073) (-33.3882, -119.4989) (-33.3927, -119.5906) (-33.3969, -119.6824) (-33.4008, -119.7743) (-33.4045, -119.8662) (-33.4071, -119.9398) (-33.409, -119.9951) (-33.4102, -120.0319) (-33.4108, -120.0504) knots 0.405839 0.405839 0.405839 0.405839 0.405839 0.405839 0.414286 0.428571 0.442857 0.457143 0.471429 0.485714 0.5 0.514286 0.528571 0.542857 0.557143 0.571429 0.585714 0.6 0.614286 0.628571 0.642857 0.657143 0.671429 0.685714 0.7 0.714286 0.728571 0.742857 0.757143 0.771429 0.785714 0.8 0.814286 0.828571 0.842857 0.857143 0.871429 0.885714 0.9 0.914286 0.928571 0.942857 0.957143 0.971429 0.985714 1 1 1 1 1 1
  arc A121 (-33.4108, -120.0504) -> (-32.2075, -120.5999) centre (-2.0032, -52.8695) ccw
  spline S121 degree 5 poles (-32.2075, -120.5999) (-32.194, -120.5873) (-32.1669, -120.5623) (-32.1264, -120.5247) (-32.0725, -120.4745) (-32.0054, -120.4115) (-31.9385, -120.3484) (-31.8719, -120.2851) (-31.8056, -120.2216) (-31.7395, -120.158) (-31.6737, -120.0942) (-31.6081, -120.0302) (-31.5428, -119.966) (-31.4777, -119.9017) (-31.4129, -119.8372) (-31.3484, -119.7725) (-31.2842, -119.7076) (-31.2202, -119.6426) (-31.1565, -119.5774) (-31.0931, -119.512) (-31.03, -119.4464) (-30.9672, -119.3807) (-30.9046, -119.3147) (-30.8423, -119.2486) (-30.7804, -119.1823) (-30.7187, -119.1159) (-30.6573, -119.0492) (-30.5962, -118.9824) (-30.5354, -118.9153) (-30.475, -118.8481) (-30.4148, -118.7807) (-30.355, -118.7131) (-30.2955, -118.6453) (-30.2363, -118.5774) (-30.1774, -118.5092) (-30.1189, -118.4408) (-30.0607, -118.3723) (-30.0028, -118.3035) (-29.9453, -118.2346) (-29.8881, -118.1654) (-29.8313, -118.096) (-29.7749, -118.0265) (-29.7234, -117.9624) (-29.6833, -117.9122) (-29.6545, -117.8758) (-29.6369, -117.8535) (-29.6304, -117.8452) knots -1 -1 -1 -1 -1 -1 -0.985714 -0.971429 -0.957143 -0.942857 -0.928571 -0.914286 -0.9 -0.885714 -0.871429 -0.857143 -0.842857 -0.828571 -0.814286 -0.8 -0.785714 -0.771429 -0.757143 -0.742857 -0.728571 -0.714286 -0.7 -0.685714 -0.671429 -0.657143 -0.642857 -0.628571 -0.614286 -0.6 -0.585714 -0.571429 -0.557143 -0.542857 -0.528571 -0.514286 -0.5 -0.485714 -0.471429 -0.457143 -0.442857 -0.428571 -0.414286 -0.405839 -0.405839 -0.405839 -0.405839 -0.405839 -0.405839
  arc A122 (-29.6304, -117.8452) -> (-28.4126, -118.3496) centre (-2.0032, -52.8695) ccw
  spline S122 degree 5 poles (-28.4126, -118.3496) (-28.4139, -118.3601) (-28.4172, -118.3884) (-28.4225, -118.4344) (-28.4298, -118.4982) (-28.4386, -118.58) (-28.4479, -118.6691) (-28.4568, -118.7583) (-28.4653, -118.8476) (-28.4734, -118.937) (-28.4811, -119.0266) (-28.4884, -119.1162) (-28.4953, -119.2059) (-28.5019, -119.2958) (-28.5081, -119.3857) (-28.514, -119.4757) (-28.5195, -119.5658) (-28.5246, -119.656) (-28.5294, -119.7463) (-28.5338, -119.8366) (-28.5379, -119.9271) (-28.5416, -120.0176) (-28.545, -120.1083) (-28.548, -120.199) (-28.5507, -120.2897) (-28.5531, -120.3806) (-28.5552, -120.4715) (-28.5569, -120.5625) (-28.5583, -120.6536) (-28.5594, -120.7447) (-28.5601, -120.836) (-28.5606, -120.9272) (-28.5607, -121.0186) (-28.5605, -121.11) (-28.56, -121.2015) (-28.5592, -121.2931) (-28.5581, -121.3847) (-28.5566, -121.4764) (-28.5549, -121.5681) (-28.5529, -121.6599) (-28.5505, -121.7518) (-28.5479, -121.8437) (-28.545, -121.9356) (-28.5424, -122.0093) (-28.5403, -122.0645) (-28.5389, -122.1014) (-28.5381, -122.1198) knots 0.405839 0.405839 0.405839 0.405839 0.405839 0.405839 0.414286 0.428571 0.442857 0.457143 0.471429 0.485714 0.5 0.514286 0.528571 0.542857 0.557143 0.571429 0.585714 0.6 0.614286 0.628571 0.642857 0.657143 0.671429 0.685714 0.7 0.714286 0.728571 0.742857 0.757143 0.771429 0.785714 0.8 0.814286 0.828571 0.842857 0.857143 0.871429 0.885714 0.9 0.914286 0.928571 0.942857 0.957143 0.971429 0.985714 1 1 1 1 1 1
  arc A123 (-28.5381, -122.1198) -> (-27.2988, -122.582) centre (-2.0032, -52.8695) ccw
  spline S123 degree 5 poles (-27.2988, -122.582) (-27.2861, -122.5686) (-27.2609, -122.5417) (-27.2232, -122.5013) (-27.173, -122.4474) (-27.1106, -122.3798) (-27.0484, -122.312) (-26.9865, -122.2441) (-26.9248, -122.1761) (-26.8634, -122.1079) (-26.8023, -122.0395) (-26.7415, -121.971) (-26.6809, -121.9024) (-26.6206, -121.8336) (-26.5606, -121.7646) (-26.5009, -121.6955) (-26.4414, -121.6262) (-26.3822, -121.5568) (-26.3234, -121.4872) (-26.2648, -121.4174) (-26.2065, -121.3475) (-26.1485, -121.2775) (-26.0908, -121.2072) (-26.0334, -121.1369) (-25.9763, -121.0663) (-25.9195, -120.9956) (-25.8631, -120.9247) (-25.8069, -120.8537) (-25.7511, -120.7825) (-25.6956, -120.7112) (-25.6404, -120.6396) (-25.5855, -120.5679) (-25.531, -120.4961) (-25.4768, -120.4241) (-25.4229, -120.3519) (-25.3694, -120.2795) (-25.3163, -120.207) (-25.2635, -120.1343) (-25.211, -120.0614) (-25.1589, -119.9883) (-25.1072, -119.9151) (-25.0559, -119.8417) (-25.0091, -119.7741) (-24.9727, -119.7211) (-24.9466, -119.6828) (-24.9306, -119.6593) (-24.9247, -119.6505) knots -1 -1 -1 -1 -1 -1 -0.985714 -0.971429 -0.957143 -0.942857 -0.928571 -0.914286 -0.9 -0.885714 -0.871429 -0.857143 -0.842857 -0.828571 -0.814286 -0.8 -0.785714 -0.771429 -0.757143 -0.742857 -0.728571 -0.714286 -0.7 -0.685714 -0.671429 -0.657143 -0.642857 -0.628571 -0.614286 -0.6 -0.585714 -0.571429 -0.557143 -0.542857 -0.528571 -0.514286 -0.5 -0.485714 -0.471429 -0.457143 -0.442857 -0.428571 -0.414286 -0.405839 -0.405839 -0.405839 -0.405839 -0.405839 -0.405839
  arc A124 (-24.9247, -119.6505) -> (-23.674, -120.0668) centre (-2.0032, -52.8695) ccw
  spline S124 degree 5 poles (-23.674, -120.0668) (-23.6745, -120.0774) (-23.6758, -120.1058) (-23.6779, -120.1521) (-23.6805, -120.2163) (-23.6836, -120.2984) (-23.6864, -120.388) (-23.6889, -120.4776) (-23.691, -120.5673) (-23.6927, -120.6571) (-23.694, -120.7469) (-23.6949, -120.8368) (-23.6955, -120.9268) (-23.6956, -121.0169) (-23.6954, -121.107) (-23.6948, -121.1972) (-23.6938, -121.2875) (-23.6925, -121.3778) (-23.6908, -121.4682) (-23.6888, -121.5587) (-23.6864, -121.6492) (-23.6837, -121.7398) (-23.6806, -121.8304) (-23.6772, -121.9211) (-23.6734, -122.0118) (-23.6693, -122.1026) (-23.6649, -122.1935) (-23.6601, -122.2844) (-23.655, -122.3753) (-23.6496, -122.4663) (-23.6438, -122.5573) (-23.6377, -122.6484) (-23.6313, -122.7396) (-23.6246, -122.8307) (-23.6176, -122.9219) (-23.6102, -123.0132) (-23.6026, -123.1045) (-23.5946, -123.1959) (-23.5864, -123.2872) (-23.5778, -123.3787) (-23.5689, -123.4701) (-23.5597, -123.5616) (-23.5502, -123.6531) (-23.5424, -123.7264) (-23.5364, -123.7813) (-23.5323, -123.818) (-23.5303, -123.8363) knots 0.405839 0.405839 0.405839 0.405839 0.405839 0.405839 0.414286 0.428571 0.442857 0.457143 0.471429 0.485714 0.5 0.514286 0.528571 0.542857 0.557143 0.571429 0.585714 0.6 0.614286 0.628571 0.642857 0.657143 0.671429 0.685714 0.7 0.714286 0.728571 0.742857 0.757143 0.771429 0.785714 0.8 0.814286 0.828571 0.842857 0.857143 0.871429 0.885714 0.9 0.914286 0.928571 0.942857 0.957143 0.971429 0.985714 1 1 1 1 1 1
  arc A125 (-23.5303, -123.8363) -> (-22.2611, -124.209) centre (-2.0032, -52.8695) ccw
  spline S125 degree 5 poles (-22.2611, -124.209) (-22.2494, -124.1947) (-22.2262, -124.166) (-22.1914, -124.1231) (-22.1453, -124.0657) (-22.0878, -123.9938) (-22.0306, -123.9218) (-21.9737, -123.8497) (-21.917, -123.7774) (-21.8607, -123.705) (-21.8046, -123.6325) (-21.7488, -123.5598) (-21.6933, -123.487) (-21.638, -123.414) (-21.5831, -123.341) (-21.5284, -123.2678) (-21.4741, -123.1944) (-21.42, -123.1209) (-21.3663, -123.0473) (-21.3128, -122.9736) (-21.2597, -122.8997) (-21.2068, -122.8257) (-21.1543, -122.7515) (-21.102, -122.6772) (-21.0501, -122.6028) (-20.9985, -122.5282) (-20.9473, -122.4535) (-20.8963, -122.3786) (-20.8457, -122.3036) (-20.7954, -122.2285) (-20.7455, -122.1532) (-20.6959, -122.0778) (-20.6466, -122.0022) (-20.5977, -121.9265) (-20.5491, -121.8507) (-20.5009, -121.7747) (-20.4531, -121.6985) (-20.4056, -121.6222) (-20.3585, -121.5458) (-20.3117, -121.4692) (-20.2654, -121.3925) (-20.2194, -121.3156) (-20.1775, -121.2448) (-20.145, -121.1894) (-20.1217, -121.1493) (-20.1075, -121.1247) (-20.1022, -121.1156) knots -1 -1 -1 -1 -1 -1 -0.985714 -0.971429 -0.957143 -0.942857 -0.928571 -0.914286 -0.9 -0.885714 -0.871429 -0.857143 -0.842857 -0.828571 -0.814286 -0.8 -0.785714 -0.771429 -0.757143 -0.742857 -0.728571 -0.714286 -0.7 -0.685714 -0.671429 -0.657143 -0.642857 -0.628571 -0.614286 -0.6 -0.585714 -0.571429 -0.557143 -0.542857 -0.528571 -0.514286 -0.5 -0.485714 -0.471429 -0.457143 -0.442857 -0.428571 -0.414286 -0.405839 -0.405839 -0.405839 -0.405839 -0.405839 -0.405839
  arc A126 (-20.1022, -121.1156) -> (-18.825, -121.4416) centre (-2.0032, -52.8695) ccw